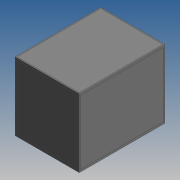
# Autodesk Inventor part: P004_CageDeTest2
Saved by Autodesk Inventor 2021.3 (Build 253353000, 353)
## iProperties
Created: 2021-09-24
Part Number: P004_CageDeTest2
Material: Générique
Document SubType Name: Modeling
Designer: gabri
Density: 1 g/cm^3
Appearance: Par défaut
Author: gabri
Autodesk Inventor part; units mm, degrees
ref_plane "YZ Plane" through (0, 0, 0) normal (1, 0, 0) x (0, 1, 0)
ref_plane "XZ Plane" through (0, 0, 0) normal (0, 1, 0) x (-1, 0, 0)
ref_plane "XY Plane" through (0, 0, 0) normal (0, 0, 1) x (1, 0, 0)
sketch "Sketch5" plane through (0, 0, 0) normal (0, 0, 1) x (1, 0, 0)
  line L0 (750, 1000) -> (-750, 1000)
  line L1 (-750, 1000) -> (-750, -1000)
  line L2 (-750, -1000) -> (750, -1000)
  line L3 (750, -1000) -> (750, 1000)
  line L4 (750, 1000) -> (-750, -1000) construction
  line L5 (-750, 1000) -> (750, -1000) construction
  line L6 (726, 976) -> (-726, 976)
  line L7 (-726, 976) -> (-726, -976)
  line L8 (-726, -976) -> (726, -976)
  line L9 (726, -976) -> (726, 976)
  line L10 (726, 976) -> (-726, -976) construction
  line L11 (-726, 976) -> (726, -976) construction
  point P0 (0, 0)
  dimension "d14" = 2000
  dimension "d15" = 1500
  dimension "d16" = 24
  dimension "d17" = 24
  constraints: 24 end point, 4 midpoint, 4 parallel, 2 horizontal, 2 perpendicular
  measures "d14" distance of L0.end L1.end
  measures "d15" distance between parallel lines of L3 L1
  measures "d16" distance between parallel lines of L1 L7
  measures "d17" distance between parallel lines of L2 L8
extrude "Extrusion4" add sketch "Sketch5" along normal blind 48
sketch "Sketch6" plane through (0, 0, 48) normal (0, 0, 1) x (1, 0, 0)
  line L0 (-750, 1000) -> (-750, -1000) construction
  line L1 (-750, -1000) -> (750, -1000) construction
  line L2 (750, -1000) -> (750, 1000) construction
  line L3 (750, 1000) -> (-750, 1000) construction
  line L4 (726, 976) -> (726, -976) construction
  line L5 (726, -976) -> (-726, -976) construction
  line L6 (-726, -976) -> (-726, 976) construction
  line L7 (-726, 976) -> (726, 976) construction
  line L8 (750, -1000) -> (702, -1000)
  line L9 (702, -1000) -> (702, -976)
  line L10 (702, -976) -> (750, -976)
  line L11 (750, -976) -> (750, -1000)
  line L12 (-750, -1000) -> (-702, -1000)
  line L13 (-702, -1000) -> (-702, -976)
  line L14 (-702, -976) -> (-750, -976)
  line L15 (-750, -976) -> (-750, -1000)
  line L16 (-750, 1000) -> (-702, 1000)
  line L17 (-702, 1000) -> (-702, 976)
  line L18 (-702, 976) -> (-750, 976)
  line L19 (-750, 976) -> (-750, 1000)
  line L20 (750, 1000) -> (702, 1000)
  line L21 (702, 1000) -> (702, 976)
  line L22 (702, 976) -> (750, 976)
  line L23 (750, 976) -> (750, 1000)
  point P0 (0, 0)
  dimension "d20" = 48
  dimension "d21" = 48
  constraints: 32 end point, 8 parallel, 6 point on line, 4 horizontal, 4 perpendicular
  measures "d20" distance of L9.end L10.end
  measures "d21" distance of L14.end L13.end
extrude "Extrusion5" add sketch "Sketch6" along normal blind 1500
sketch "Sketch7" plane through (0, 0, 1548) normal (0, 0, 1) x (1, 0, 0)
  line L0 (-702, -976) -> (-702, -1000) construction
  line L1 (-702, -1000) -> (702, -1000) construction
  line L2 (702, -1000) -> (702, -976) construction
  line L3 (702, -976) -> (-702, -976) construction
  line L4 (-726, 976) -> (-750, 976) construction
  line L5 (-750, 976) -> (-750, -976) construction
  line L6 (-750, -976) -> (-726, -976) construction
  line L7 (-726, -976) -> (-726, 976) construction
  line L8 (702, 1000) -> (702, 976) construction
  line L9 (702, 976) -> (750, 976) construction
  line L10 (750, 976) -> (750, 1000) construction
  line L11 (750, 1000) -> (702, 1000) construction
  line L12 (750, 1000) -> (-750, 1000)
  line L13 (-750, 1000) -> (-750, -1000)
  line L14 (-750, -1000) -> (750, -1000)
  line L15 (750, -1000) -> (750, 1000)
  line L16 (-726, -976) -> (726, -976)
  line L17 (726, -976) -> (726, 976)
  line L18 (726, 976) -> (-726, 976)
  line L19 (-726, 976) -> (-726, -976)
  point P0 (0, 0)
  dimension "d24" = 24
  constraints: 16 end point, 4 parallel, 2 horizontal, 2 perpendicular, 1 midpoint
  measures "d24" distance between parallel lines of L3 L14
extrude "Extrusion6" add sketch "Sketch7" along normal blind 48
sketch "Sketch8" plane through (750, -1000, 0) normal (1, 0, 0) x (0, 0, -1)
  line L0 (-48, 1976) -> (-1548, 1976) construction
  line L1 (-48, 24) -> (-48, 1976) construction
  line L2 (-48, 24) -> (-1548, 24) construction
  line L3 (-1548, 24) -> (-1548, 1976) construction
  line L4 (0, 2000) -> (-1596, 2000) construction
  line L5 (-1596, 0) -> (-1596, 2000) construction
  line L6 (0, 0) -> (-1596, 0) construction
  line L7 (0, 0) -> (0, 2000) construction
  line L8 (-1596, 0) -> (0, 0)
  line L9 (0, 0) -> (0, 2000)
  line L10 (0, 2000) -> (-1596, 2000)
  line L11 (-1596, 2000) -> (-1596, 0)
  point P0 (0, 1000)
  constraints: 8 end point, 2 parallel, 1 horizontal, 1 perpendicular
extrude "Extrusion7" add sketch "Sketch8" along normal blind 0.1
sketch "Sketch9" plane through (-750, -1000, 0) normal (0, -1, 0) x (1, 0, 0)
  line L0 (1452, 48) -> (1452, 1548) construction
  line L1 (48, 48) -> (1452, 48) construction
  line L2 (48, 48) -> (48, 1548) construction
  line L3 (48, 1548) -> (1452, 1548) construction
  line L4 (0, 1596) -> (1500.1, 1596) construction
  line L5 (0, 0) -> (0, 1596) construction
  line L6 (0, 0) -> (1500.1, 0) construction
  line L7 (1500.1, 1596) -> (1500.1, 0) construction
  line L8 (0, 1596) -> (1500.1, 1596)
  line L9 (1500.1, 1596) -> (1500.1, 0)
  line L10 (1500.1, 0) -> (0, 0)
  line L11 (0, 0) -> (0, 1596)
  point P0 (750, 0)
  constraints: 8 end point, 2 parallel, 1 horizontal, 1 perpendicular
extrude "Extrusion8" add sketch "Sketch9" along normal blind 0.1
sketch "Sketch10" plane through (-750, 1000, 0) normal (-1, 0, 0) x (0, 0, 1)
  line L0 (0, 0) -> (1596, 0) construction
  line L1 (0, 0) -> (0, -2000.1) construction
  line L2 (1596, -2000.1) -> (0, -2000.1) construction
  line L3 (1596, 0) -> (1596, -2000.1) construction
  line L4 (1548, -24) -> (1548, -1976) construction
  line L5 (48, -1976) -> (1548, -1976) construction
  line L6 (48, -24) -> (48, -1976) construction
  line L7 (48, -24) -> (1548, -24) construction
  line L8 (1596, 0) -> (0, 0)
  line L9 (0, 0) -> (0, -2000.1)
  line L10 (0, -2000.1) -> (1596, -2000.1)
  line L11 (1596, -2000.1) -> (1596, 0)
  line L12 (1348, -700) -> (1048, -700)
  line L13 (1048, -700) -> (1048, -1300)
  line L14 (1048, -1300) -> (1348, -1300)
  line L15 (1348, -1300) -> (1348, -700)
  line L16 (-319.34, -1000) -> (1915.34, -1000) construction
  point P0 (0, -1000)
  dimension "d37" = 600
  dimension "d38" = 300
  dimension "d39" = 300
  dimension "d40" = 1000
  constraints: 16 end point, 4 parallel, 2 horizontal, 2 perpendicular
  measures "d37" distance between parallel lines of L14 L12
  measures "d38" distance between parallel lines of L13 L15
  measures "d39" distance between parallel lines of L16 L12
  measures "d40" distance between parallel lines of L6 L13
extrude "Extrusion9" add sketch "Sketch10" along normal blind 0.1
sketch "Sketch11" plane through (0, 0, 1596) normal (0, 0, 1) x (1, 0, 0)
  line L0 (750.1, -1000.1) -> (-750.1, -1000.1) construction
  line L1 (750.1, 1000) -> (750.1, -1000.1) construction
  line L2 (-750.1, 1000) -> (750.1, 1000) construction
  line L3 (-750.1, -1000.1) -> (-750.1, 1000) construction
  line L4 (-726, -976) -> (-726, 976) construction
  line L5 (-726, 976) -> (726, 976) construction
  line L6 (726, 976) -> (726, -976) construction
  line L7 (726, -976) -> (-726, -976) construction
  line L8 (750.1, 1000) -> (-750.1, 1000)
  line L9 (-750.1, 1000) -> (-750.1, -1000.1)
  line L10 (-750.1, -1000.1) -> (750.1, -1000.1)
  line L11 (750.1, -1000.1) -> (750.1, 1000)
  point P0 (0, 0)
  constraints: 8 end point, 2 parallel, 1 horizontal, 1 perpendicular
extrude "Extrusion10" add sketch "Sketch11" along normal blind 0.1
sketch "Sketch12" plane through (0, 0, 0) normal (0, 0, -1) x (-1, 0, 0)
  line L0 (750.1, 1000) -> (-750.1, 1000) construction
  line L1 (-750.1, 1000) -> (-750.1, -1000.1) construction
  line L2 (-750.1, -1000.1) -> (750.1, -1000.1) construction
  line L3 (750.1, 1000) -> (750.1, -1000.1) construction
  line L4 (-726, 976) -> (-726, -976) construction
  line L5 (726, 976) -> (-726, 976) construction
  line L6 (726, -976) -> (726, 976) construction
  line L7 (-726, -976) -> (726, -976) construction
  line L8 (750.1, 1000) -> (-750.1, 1000)
  line L9 (-750.1, 1000) -> (-750.1, -1000.1)
  line L10 (-750.1, -1000.1) -> (750.1, -1000.1)
  line L11 (750.1, -1000.1) -> (750.1, 1000)
  point P0 (0, 0)
  constraints: 8 end point, 2 parallel, 1 horizontal, 1 perpendicular
extrude "Extrusion11" add sketch "Sketch12" along normal blind 0.1
sketch "Sketch13" plane through (-750.1, 1000, 1596.1) normal (0, 1, 0) x (1, 0, 0)
  line L0 (48.1, 1548.1) -> (48.1, 48.1) construction
  line L1 (1452.1, 1548.1) -> (48.1, 1548.1) construction
  line L2 (1452.1, 1548.1) -> (1452.1, 48.1) construction
  line L3 (1452.1, 48.1) -> (48.1, 48.1) construction
  line L4 (1500.2, 0) -> (1500.2, 1596.2) construction
  line L5 (0, 1596.2) -> (1500.2, 1596.2) construction
  line L6 (0, 1596.2) -> (0, 0) construction
  line L7 (1500.2, 0) -> (0, 0) construction
  line L8 (0, 0) -> (1500.2, 1596.2)
  line L9 (1500.2, 0) -> (1500.2, 1596.2)
  line L10 (1500.2, 0) -> (0, 0)
  point P0 (750.1, 1596.1)
  constraints: 6 end point, 1 collinear, 1 perpendicular
extrude "Extrusion12" add sketch "Sketch13" along normal blind 0.1
body "Solid2"
